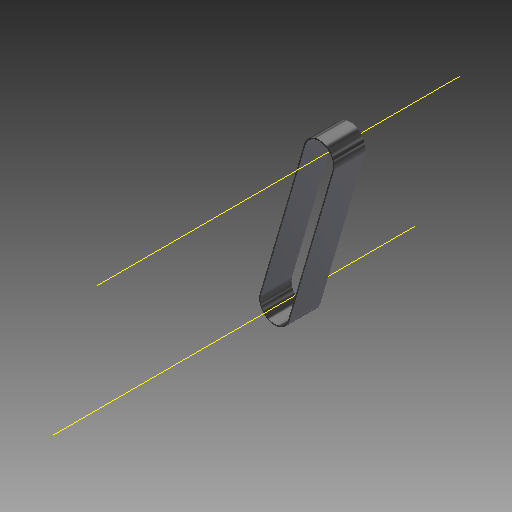
# Autodesk Inventor part: Synchronous Belt
Saved by Autodesk Inventor 2019.4 (Build 234330000, 330)
## iProperties
Created: 2020-01-11
Part Number: Synchronous Belt
Material: Rubber
Document SubType Name: Modeling
Designer: admin
Density: 0.93 g/cm^3
Appearance: Rubber - Black - Version 1.1
Mass: 7.6725 g
Surface Area: 171.6 cm^2
Volume: 8.25 cm^3
CustomPartVersion: 1
Author: admin
Autodesk Inventor part; units mm, degrees
sketch "Sketch Path" plane through (0, 0, 0) normal (0, 0, 1) x (1, 0, 0)
  arc A0 (180.4294, 217.4975) -> (157.517, 224.2023) centre (168.9732, 220.8499) ccw
  arc A1 (121.7086, 101.834) -> (144.621, 95.1292) centre (133.1648, 98.4816) ccw
  line L0 (121.7086, 101.834) -> (157.517, 224.2023)
  line L1 (180.4294, 217.4975) -> (144.621, 95.1292)
  constraints: 4 end point, 4 point on circle, 2 centre point
ref_plane "Cross Section Plane" through (157.517, 224.2023, 0) normal (-0.2808, -0.9598, 0) x (0, 0, 1)
ref_plane "Work Plane2" through (168.9732, 220.8499, 0) normal (-1, 0, 0) x (0, 0, 1)
ref_plane "Work Plane3" through (133.1648, 98.4816, 0) normal (0.309, 0.9511, 0) x (0, 0, 1)
sketch "Cross Section" plane through (157.517, 224.2023, 0) normal (-0.2808, -0.9598, 0) x (0, 0, 1)
  line L0 (-12.5, 0.5) -> (12.5, 0.5)
  line L1 (12.5, 0.5) -> (12.5, -0.5)
  line L2 (12.5, -0.5) -> (-12.5, -0.5)
  line L3 (-12.5, -0.5) -> (-12.5, 0.5)
  line L4 (-12.5, 0) -> (12.5, 0) construction
  point P0 (0, 0)
  point P1 (0, 0)
  dimension "d0" = 25
  dimension "d4" = 0.5
  dimension "d5" = 0.5
  constraints: 10 end point, 3 midpoint, 2 parallel, 1 coincident, 1 horizontal, 1 perpendicular, 1 other
  measures "d0" distance between parallel lines of L1 L3
  measures "d4" distance between parallel lines of L2 L4
  measures "d5" distance between parallel lines of L4 L0
sweep "Belt" add profiles "Cross Section" path "Sketch Path"
equation "\"d0\" = da_B"
equation "\"d4\" = da_a"
equation "\"d5\" = da_a2"
equation "\"da_B\" = 25"
equation "\"da_pb\" = 5"
equation "\"da_a\" = 0.5"
equation "\"da_S\" = 2.65"
equation "\"da_Beta\" = 20deg"
equation "\"da_Ht\" = 1.2"
equation "\"da_H\" = 2.2"
equation "\"da_a2\" = 0.5"
body "Solid1"
